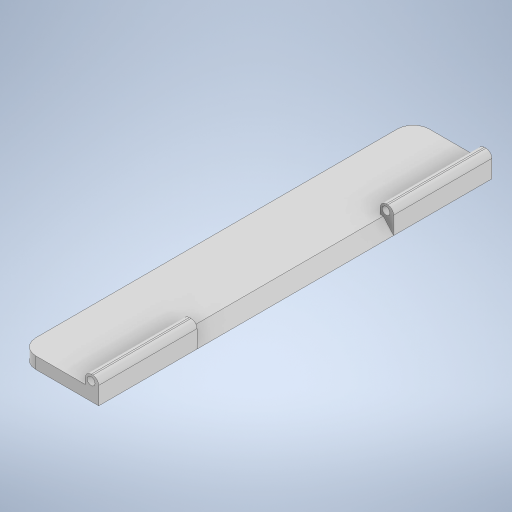
# Autodesk Inventor part: Cover
Saved by Autodesk Inventor 2023 (Build 270158000, 158)
## iProperties
Created: 2023-03-07
Part Number: Cover
Material: Типовые
Document SubType Name: Modeling
Designer: Josh
Density: 1 g/cm^3
Appearance: По умолчанию
Author: Josh
Autodesk Inventor part; units mm, degrees
ref_plane "YZ Plane" through (0, 0, 0) normal (1, 0, 0) x (0, 1, 0)
ref_plane "XZ Plane" through (0, 0, 0) normal (0, 1, 0) x (-1, 0, 0)
ref_plane "XY Plane" through (0, 0, 0) normal (0, 0, 1) x (1, 0, 0)
sketch "Эскиз2" plane through (0, 0, 0) normal (0, 0, 1) x (1, 0, 0)
  line L0 (0, 0) -> (20, 0)
  line L1 (20, 0) -> (20, 3)
  line L2 (20, 3) -> (0, 3)
  line L3 (0, 3) -> (0, 0)
  dimension "d14" = 20
  dimension "d15" = 3
  constraints: 8 end point, 2 parallel, 1 horizontal, 1 perpendicular
  measures "d14" distance between parallel lines of L3 L1
  measures "d15" distance between parallel lines of L0 L2
extrude "Выдавливание2" add sketch "Эскиз2" along normal mid plane 100
fillet "Сопряжение1" radius 4 2 edges at (0, 1.5, 50) (0, 1.5, -50)
sketch "Эскиз5" plane through (20, 3, 50) normal (0, 1, 0) x (1, 0, 0)
  line L0 (0, 100) -> (0, 0) projected
  line L1 (0, 0) -> (-16, 0) projected
  line L2 (0, 100) -> (-3.42, 100)
  line L3 (-3.42, 100) -> (-3.42, 0)
  line L4 (-3.42, 0) -> (0, 0)
  line L5 (0, 0) -> (0, 100)
  point P0 (-20, 50)
  dimension "d25" = 3.42
  constraints: 8 end point, 2 parallel, 1 horizontal, 1 perpendicular, 1 point on line
  measures "d25" distance between parallel lines of L0 L3
extrude "Выдавливание4" add sketch "Эскиз5" along normal blind 3
sketch "Эскиз6" plane through (0, 0, 50) normal (0, 0, 1) x (1, 0, 0)
  circle A0 centre (18.08, 4.5) radius 1
  line L0 (16.58, 6) -> (20, 6) projected
  line L1 (16.58, 3) -> (16.58, 6) projected
  point P0 (0, 0)
  dimension "d28" = 2
  dimension "d29" = 1.5
  dimension "d30" = 1.5
  constraints: 1 centre point
  measures "d28" diameter of A0
  measures "d29" distance from line of A0.centre L0
  measures "d30" distance from line of L1 A0.centre
extrude "Выдавливание5" cut sketch "Эскиз6" against normal through all
sketch "Эскиз7" plane through (20, 6, 50) normal (0, 1, 0) x (1, 0, 0)
  line L0 (-3.42, 100) -> (-3.42, 0) projected
  line L1 (0, 0) -> (0, 100) projected
  line L2 (-3.42, 25) -> (0, 25)
  line L3 (0, 25) -> (0, 75)
  line L4 (0, 75) -> (-3.42, 75)
  line L5 (-3.42, 75) -> (-3.42, 25)
  line L6 (-3.42, 0) -> (-16, 0) projected
  point P0 (-20, 50)
  point P1 (-3.42, 75)
  point P2 (0, 25)
  dimension "d33" = 50
  dimension "d34" = 25
  constraints: 8 end point, 2 parallel, 2 point on line, 1 horizontal, 1 perpendicular
  measures "d33" distance between parallel lines of L2 L4
  measures "d34" distance between parallel lines of L6 L2
extrude "Выдавливание6" cut sketch "Эскиз7" against normal blind 3
fillet "Сопряжение2" radius 1.5 4 edges at (20, 6, 37.5) (16.58, 6, 37.5) (20, 6, -37.5) (16.58, 6, -37.5)
sketch "Эскиз8" plane through (16.58, 3, -25) normal (0, 0, 1) x (1, 0, 0)
  line L0 (3.42, -3) -> (3.42, 1.5) projected
  line L1 (0, 0.9343) -> (3.42, -3)
  line L2 (3.42, -3) -> (-12.58, -3) projected
  line L3 (0, 0) -> (0, 1.5) projected
  line L4 (0, 0.9343) -> (3.42, 0.9343)
  point P0 (-16.58, -3)
  dimension "d38" = 49
  constraints: 4 end point, 2 point on line, 1 perpendicular
  measures "d38" angle of L2 L1
extrude "Выдавливание7" cut sketch "Эскиз8" along normal up to surface (50 mm away)
